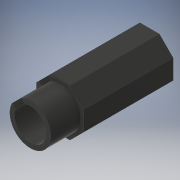
# Autodesk Inventor part: conduit_endcap
Saved by Autodesk Inventor 2017 (Build 210142000, 142)
## iProperties
Created: 2018-11-30
Part Number: conduit_endcap
Material: UHMW, Black
Document SubType Name: Modeling
Designer: ddeboer
Density: 0.94 g/cm^3
Appearance: Smooth - Black
Author: ddeboer
Autodesk Inventor part; units mm, degrees
ref_plane "YZ Plane" through (0, 0, 0) normal (1, 0, 0) x (0, 1, 0)
ref_plane "XZ Plane" through (0, 0, 0) normal (0, 1, 0) x (-1, 0, 0)
ref_plane "XY Plane" through (0, 0, 0) normal (0, 0, 1) x (1, 0, 0)
sketch "Sketch1" plane through (0, 0, 0) normal (0, 0, 1) x (1, 0, 0)
  arc A0 (0, 8) -> (0, -8) centre (0, 0) ccw
  line L0 (0, 8) -> (0, 19.75)
  line L1 (0, -8) -> (0, -19.75)
  line L2 (0, -19.75) -> (-8.18, -19.75)
  line L3 (0, 19.75) -> (-8.18, 19.75)
  line L4 (-8.18, 19.75) -> (-19.7497, 8.1803)
  line L5 (-8.18, 19.75) -> (8.182, 19.75) construction
  line L6 (-19.7497, 8.1803) -> (-19.7497, -8.1797)
  line L7 (-19.7497, 8.1803) -> (-3.3897, 8.1803) construction
  line L8 (-19.7497, -8.1797) -> (-8.18, -19.75)
  dimension "d0" = 16
  dimension "d1" = 11.75
  dimension "d2" = 11.75
  dimension "d3" = 8.18
  dimension "d4" = 8.18
  dimension "d5" = 16.362
  dimension "d6" = 135
  dimension "d9" = 16.36
  dimension "d10" = 90
  constraints: 18 end point, 4 horizontal, 3 vertical, 2 equal length, 2 point on circle, 1 centre point, 1 coincident
  measures "d0" diameter of A0
  measures "d1" distance of L0.start L0.end
  measures "d2" distance of L1.start L1.end
  measures "d3" distance of L1.end L2.end
  measures "d4" distance of L0.end L3.end
  measures "d5" distance of L3.end L4.end
  measures "d6" angle of L4 L5
  measures "d9" distance of L4.end L6.end
  measures "d10" angle of L6 L7
extrude "Extrusion1" add sketch "Sketch1" along normal blind 100
mirror "Mirror1" about plane through (0, 8, 0) normal (1, 0, 0) of "Extrusion1"
sketch "Sketch3" plane through (0, 0, 0) normal (0, 0, -1) x (-1, 0, 0)
  circle A0 centre (0, 0) radius 13.4
  dimension "d16" = 26.8
  constraints: 1 centre point, 1 coincident
  measures "d16" diameter of A0
extrude "Extrusion3" cut sketch "Sketch3" against normal blind 110
sketch "Sketch4" plane through (0, 0, 0) normal (0, 0, -1) x (-1, 0, 0)
  circle A0 centre (0, 0) radius 16.7
  dimension "d19" = 33.4
  constraints: 1 centre point, 1 coincident
  measures "d19" diameter of A0
extrude "Extrusion4" cut sketch "Sketch4" against normal blind 10
sketch "Sketch5" plane through (0, 0, 100) normal (0, 0, 1) x (1, 0, 0)
  circle A0 centre (0, 0) radius 17.2
  circle A1 centre (0, 0) radius 24.3245
  dimension "d22" = 34.4
  constraints: 2 centre point, 2 coincident
  measures "d22" diameter of A0
extrude "Extrusion5" cut sketch "Sketch5" against normal blind 25
sketch "Sketch6" plane through (0, 0, 0) normal (0, 0, -1) x (-1, 0, 0)
  line L0 (-0.855, -8.707) -> (20.3583, 12.5062)
  line L1 (20.3583, 12.5062) -> (12.5801, 20.2844)
  line L2 (12.5801, 20.2844) -> (-8.6331, -0.9288)
  line L3 (-8.6331, -0.9288) -> (-0.855, -8.707)
  point P0 (0, 0)
  dimension "d25" = 11
  dimension "d26" = 30
  constraints: 8 end point, 2 parallel, 1 perpendicular
  measures "d25" distance of L0.end L1.end
  measures "d26" distance of L1.end L2.end
extrude "Extrusion6" cut sketch "Sketch6" against normal blind 200
body "Solid1"
